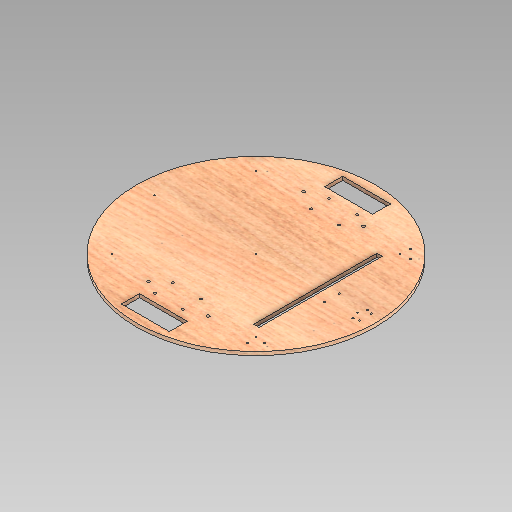
# Autodesk Inventor part: Robot_base
Saved by Autodesk Inventor 2020 (Build 240168000, 168)
## iProperties
Created: 2022-08-06
Part Number: Robot_base
Material: Birch
Document SubType Name: Modeling
Designer: umair_maher
Density: 0.512 g/cm^3
Appearance: Birch - Natural Medium Gloss
Author: umair_maher
Autodesk Inventor part; units mm, degrees
ref_plane "YZ Plane" through (0, 0, 0) normal (1, 0, 0) x (0, 1, 0)
ref_plane "XZ Plane" through (0, 0, 0) normal (0, 1, 0) x (-1, 0, 0)
ref_plane "XY Plane" through (0, 0, 0) normal (0, 0, 1) x (1, 0, 0)
sketch "Sketch1" plane through (0, 0, 0) normal (0, 1, 0) x (-1, 0, 0)
  circle A0 centre (0, 0) radius 200
  line L0 (0, 0) -> (0, -19)
  line L1 (0, 0) -> (0, -200)
  line L2 (0, -200) -> (0, -185)
  line L3 (0, -185) -> (-40, -185)
  line L4 (-40, -185) -> (40, -185)
  line L5 (40, -185) -> (40, -155)
  line L6 (40, -155) -> (-40, -155)
  line L7 (-40, -155) -> (-40, -185)
  line L8 (0, -185) -> (0, -155)
  line L9 (0, -155) -> (0, -170)
  line L10 (0, -170) -> (0, -178.5)
  line L11 (0, -178.5) -> (0, -162.5)
  line L12 (0, -178.5) -> (0, -161.5)
  line L13 (0, -178.5) -> (0, -152.5)
  line L14 (0, -152.5) -> (0, -100.5)
  line L15 (0, -100.5) -> (0, -111.5)
  line L16 (0, -111.5) -> (0, -141.5)
  line L17 (0, -111.5) -> (62.5795, -111.5)
  line L18 (62.5795, -111.5) -> (-81.3818, -111.5)
  line L19 (0, -141.5) -> (67.2407, -141.5)
  line L20 (67.2407, -141.5) -> (-91.5277, -141.5)
  line L21 (0, -111.5) -> (19.187, -111.5)
  line L22 (19.187, -111.5) -> (-27.813, -111.5)
  line L23 (-27.813, -111.5) -> (-27.813, -148.582)
  line L24 (19.187, -111.5) -> (19.187, -155)
  circle A1 centre (19.187, -111.5) radius 2
  circle A2 centre (19.187, -141.5) radius 2
  circle A3 centre (-27.813, -111.5) radius 2
  circle A4 centre (-27.813, -141.5) radius 2
  line L25 (0, 0) -> (124.6952, 0)
  circle A5 centre (0, 0) radius 1
  circle A6 centre (-154.7094, 0) radius 1
  circle A7 centre (178.175, 0) radius 1
  line L26 (0, 185) -> (-40, 185)
  line L27 (-40, 185) -> (40, 185)
  line L28 (40, 185) -> (40, 155)
  line L29 (40, 155) -> (-40, 155)
  line L30 (-40, 155) -> (-40, 185)
  line L31 (0, 185) -> (0, 155)
  line L32 (0, 155) -> (0, 170)
  line L33 (0, 170) -> (0, 178.5)
  line L34 (0, 178.5) -> (0, 162.5)
  line L35 (0, 178.5) -> (0, 161.5)
  line L36 (0, 178.5) -> (0, 152.5)
  circle A8 centre (-19.187, 111.5) radius 2
  circle A9 centre (-19.187, 141.5) radius 2
  line L37 (27.813, 141.5) -> (-19.187, 141.5)
  line L38 (-19.187, 111.5) -> (27.813, 111.5)
  circle A10 centre (27.813, 111.5) radius 2
  circle A11 centre (27.813, 141.5) radius 2
  line L39 (27.813, 141.5) -> (27.813, 111.5)
  line L40 (-19.187, 141.5) -> (-19.187, 111.5)
  line L41 (0, 0) -> (0, 200)
  line L42 (0, -100.5) -> (0, 0)
  line L43 (0, 0) -> (0, 111.5)
  dimension "d0" = 400
  dimension "d2" = 15
  dimension "d3" = 40
  dimension "d4" = 80
  dimension "d5" = 30
  dimension "d6" = 80
  dimension "d7" = 8.5
  dimension "d8" = 17
  dimension "d9" = 26
  dimension "d10" = 52
  dimension "d15" = 4
  dimension "d16" = 4
  dimension "d17" = 4
  dimension "d18" = 4
  dimension "d21" = 2
  dimension "d22" = 2
  dimension "d23" = 2
  dimension "d35" = 47
  dimension "d36" = 30
  dimension "d37" = 19.187
  dimension "d38" = 11
  dimension "d39" = 4
  dimension "d40" = 47
  dimension "d41" = 30
  dimension "d42" = 111.5
  dimension "d43" = 19.187
  constraints: 88 end point, 23 point on line, 12 centre point, 11 symmetric about line, 6 coincident, 6 perpendicular, 4 vertical, 3 horizontal, 3 midpoint, 2 point on circle, 1 collinear
  measures "d0" diameter of A0
  measures "d2" distance of L1.end L2.end
  measures "d3" distance of L2.end L3.end
  measures "d4" distance of L3.end L4.end
  measures "d5" distance of L4.end L5.end
  measures "d6" distance of L5.end L6.end
  measures "d7" distance of L9.end L10.end
  measures "d8" distance of L10.end L12.end
  measures "d9" distance of L10.end L13.end
  measures "d10" distance of L13.end L14.end
  measures "d15" diameter of A1
  measures "d16" diameter of A2
  measures "d17" diameter of A3
  measures "d18" diameter of A4
  measures "d21" diameter of A5
  measures "d22" diameter of A6
  measures "d23" diameter of A7
  measures "d35" distance between parallel lines of L23 L24
  measures "d36" distance between parallel lines of L20 L22
  measures "d37" distance between parallel lines of L1 L24
  measures "d38" distance from line of L18 L14.end
  measures "d39" diameter of A11
  measures "d40" distance between parallel lines of L40 L39
  measures "d41" distance between parallel lines of L38 L37
  measures "d42" distance of point (0, 0) L43.end
  measures "d43" distance between parallel lines of L40 L41
extrude "Extrusion1" add sketch "Sketch1" along normal blind 6 contours A0 L1 L4 L5 L6 L24 A2 A1 L17 L0 A5 L41 L38 A10 L39 A11 L37 L36 L29 L28 L27 | L41 L26 L30 L29 L36 L37 A9 L40 A8 L38 A5 L0 L1 L18 A3 L23 A4 L20 L6 L7 L3 A0 | L1 L19 A2 L24 L6 | L41 L38 A8 L40 A9 L37 | L37 A11 L39 A10 L38 L41 | L20 A4 L23 A3 L18 L1 | L1 L17 A1 L24 A2 L19 | A6 | A7
sketch "Sketch2" plane through (0, 6, 0) normal (0, 1, 0) x (1, 0, 0)
  circle A0 centre (0, 0) radius 1 projected
  line L0 (0, 0) -> (233.037, 233.037)
  line L1 (0, 0) -> (329.564, 0) construction
  line L2 (0, 0) -> (120.2082, 120.2082)
  circle A1 centre (120.2082, 120.2082) radius 1
  dimension "d24" = 45
  dimension "d25" = 170
  dimension "d26" = 2
  constraints: 6 end point, 1 centre point, 1 coincident, 1 equal length, 1 horizontal, 1 point on line
  measures "d24" angle of L1 L0
  measures "d25" distance of L0.start L2.end
  measures "d26" diameter of A1
extrude "Extrusion2" cut sketch "Sketch2" against normal blind 6 contours A1 L0 | L0 A1
pattern_circular "Circular Pattern1" count 8 over 360 about axis through (0, -10, 0) along (0, -1, 0) of "Extrusion2"
sketch "Sketch3" plane through (0, 6, 0) normal (0, 1, 0) x (1, 0, 0)
  circle A0 centre (0, 0) radius 1 projected
  line L0 (0, 0) -> (200, 0)
  circle A1 centre (0, 0) radius 200 projected
  line L1 (0, 0) -> (0, 398.337)
  line L2 (0, 398.337) -> (0, -304.2315)
  line L3 (0, 0) -> (-272.9704, 0)
  line L4 (200, 0) -> (174.2263, 0)
  line L5 (174.2263, 0) -> (174.2263, 12)
  line L6 (174.2263, 12) -> (127.2263, 12)
  line L7 (127.2263, 12) -> (127.2263, -12)
  line L8 (127.2263, -12) -> (174.2263, -12)
  line L9 (174.2263, -12) -> (174.2263, 12)
  circle A2 centre (127.2263, -12) radius 1.5
  circle A3 centre (127.2263, 12) radius 1.5
  circle A4 centre (174.2263, -12) radius 1.5
  circle A5 centre (174.2263, 12) radius 1.5
  dimension "d44" = 12
  dimension "d45" = 47
  dimension "d46" = 24
  dimension "d47" = 3
  dimension "d48" = 3
  dimension "d49" = 3
  dimension "d50" = 3
  constraints: 20 end point, 5 perpendicular, 4 centre point, 4 coincident, 3 point on line, 2 horizontal, 1 horizontal alignment, 1 vertical, 1 other
  measures "d44" distance of L4.end L5.end
  measures "d45" distance of L5.end L6.end
  measures "d46" distance of L6.end L7.end
  measures "d47" diameter of A2
  measures "d48" diameter of A3
  measures "d49" diameter of A4
  measures "d50" diameter of A5
extrude "Extrusion3" cut sketch "Sketch3" against normal blind 6 contours A3 L6 L7 | L7 L6 A3 | A2 L8 L7 | L7 L8 A2 | A5 L6 L5 | L5 L6 A5 | A4 L8 L9 | L9 L8 A4
sketch "Sketch5" plane through (0, 6, 0) normal (0, 1, 0) x (1, 0, 0)
  circle A0 centre (0, 0) radius 200 projected
  line L0 (200, 0) -> (183, 0)
  line L1 (183, 0) -> (183, 10)
  line L2 (183, 10) -> (183, 0)
  line L3 (183, 0) -> (183, -10)
  circle A1 centre (183, -10) radius 1.5
  circle A2 centre (183, 10) radius 1.5
  dimension "d53" = 17
  dimension "d54" = 10
  dimension "d55" = 10
  dimension "d56" = 10
  dimension "d57" = 3
  dimension "d58" = 3
  constraints: 8 end point, 2 centre point, 2 coincident, 1 collinear, 1 horizontal, 1 horizontal alignment, 1 perpendicular, 1 point on line, 1 other
  measures "d53" distance of L0.start L0.end
  measures "d54" distance of L0.end L1.end
  measures "d55" distance of L1.end L0.end
  measures "d56" distance of L0.end L3.end
  measures "d57" diameter of A1
  measures "d58" diameter of A2
extrude "Extrusion4" cut sketch "Sketch5" against normal blind 6 contours A1 | A2
pattern_circular "Circular Pattern2" count 2 over 45 about axis through (0, -10, 0) along (0, 1, 0) of "Extrusion4"
pattern_circular "Circular Pattern3" count 2 over 45 about axis through (0, -10, 0) along (0, -1, 0) of "Extrusion4"
sketch "Sketch6" plane through (0, 6, 0) normal (0, 1, 0) x (1, 0, 0)
  circle A0 centre (0, 0) radius 1 projected
  line L0 (0, 0) -> (0, -130)
  line L1 (-40, -155) -> (40, -155) projected
  line L2 (0, -130) -> (0, 130)
  line L3 (100.075, -103.9398) -> (109.075, -103.9398)
  line L4 (109.075, -103.9398) -> (109.075, 102.0602)
  line L5 (109.075, 102.0602) -> (100.075, 102.0602)
  line L6 (100.075, 102.0602) -> (100.075, -103.9398)
  line L7 (100.075, -103.9398) -> (109.075, 102.0602) construction
  line L8 (109.075, -103.9398) -> (100.075, 102.0602) construction
  line L9 (100.075, 102.0602) -> (70.075, 102.0602)
  line L10 (70.075, 102.0602) -> (70.075, 57.0602)
  line L11 (70.075, 57.0602) -> (94.075, 57.0602)
  line L12 (94.075, 57.0602) -> (33.1028, 57.0602)
  line L13 (33.1028, 57.0602) -> (33.1028, -101.9398)
  line L14 (33.1028, -101.9398) -> (94.075, -101.9398)
  line L15 (94.075, -101.9398) -> (94.075, 57.0602)
  line L16 (0, -155) -> (0, -85)
  line L17 (0, -85) -> (-56.011, -85)
  line L18 (-56.011, -85) -> (54.9913, -85)
  line L19 (40, 155) -> (-40, 155) projected
  line L20 (0, 155) -> (0, 85)
  line L21 (0, 85) -> (-43.3575, 85)
  line L22 (-43.3575, 85) -> (43.7057, 85)
  line L23 (-50, -130) -> (50, -130)
  line L24 (50, -130) -> (50, 130)
  line L25 (50, 130) -> (-50, 130)
  line L26 (-50, 130) -> (-50, -130)
  circle A1 centre (0, 0) radius 1 projected
  line L27 (-50, -130) -> (50, 130) construction
  line L28 (50, -130) -> (-50, 130) construction
  circle A2 centre (-50, -130) radius 2.5
  circle A3 centre (-50, 130) radius 2.5
  circle A4 centre (50, 130) radius 2.5
  circle A5 centre (50, -130) radius 2.5
  dimension "d68" = 130
  dimension "d69" = 260
  dimension "d70" = 9
  dimension "d71" = 206
  dimension "d73" = 30
  dimension "d74" = 45
  dimension "d75" = 70
  dimension "d76" = 70
  dimension "d79" = 100
  dimension "d80" = 260
  dimension "d81" = 5
  dimension "d82" = 5
  dimension "d83" = 5
  dimension "d84" = 5
  constraints: 54 end point, 8 perpendicular, 7 point on line, 4 centre point, 4 horizontal, 4 midpoint, 4 parallel, 3 coincident, 1 vertical
  measures "d68" distance of L0.start L0.end
  measures "d69" distance of L0.end L2.end
  measures "d70" distance of L5.end L4.end
  measures "d71" distance of L4.end L3.end
  measures "d73" distance of L5.end L9.end
  measures "d74" distance of L9.end L10.end
  measures "d75" distance of L16.start L16.end
  measures "d76" distance of L20.start L20.end
  measures "d79" distance of L25.end L24.end
  measures "d80" distance of L24.end L23.end
  measures "d81" diameter of A2
  measures "d82" diameter of A3
  measures "d83" diameter of A4
  measures "d84" diameter of A5
extrude "Extrusion5" cut sketch "Sketch6" against normal blind 9 contours A0 L0 L2 | L2 L0 A0 | L5 L4 L3 L6 | A3 L26 L25 | L25 L26 A3 | A4 L24 L25 | L25 L24 A4 | A2 L26 L23 | L23 L26 A2 | A5 L24 L23 | L23 L24 A5
body "Solid1"
